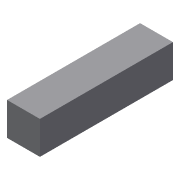
# Autodesk Inventor part: carbide_insert
Saved by Autodesk Inventor 2019 (Build 230136000, 136)
## iProperties
Created: 2023-02-17
Part Number: carbide_insert
Material: Generic
Document SubType Name: Modeling
Designer: prich
Density: 1 g/cm^3
Appearance: Default
Author: prich
Autodesk Inventor part; units mm, degrees
ref_plane "YZ Plane" through (0, 0, 0) normal (1, 0, 0) x (0, 1, 0)
ref_plane "XZ Plane" through (0, 0, 0) normal (0, 1, 0) x (-1, 0, 0)
ref_plane "XY Plane" through (0, 0, 0) normal (0, 0, 1) x (1, 0, 0)
sketch "Sketch1" plane through (0, 0, 0) normal (0, 0, 1) x (1, 0, 0)
  line L0 (0, 0) -> (1.6002, 0)
  line L1 (1.6002, 0) -> (1.6002, 1.6002)
  line L2 (1.6002, 1.6002) -> (0, 1.6002)
  line L3 (0, 1.6002) -> (0, 0)
  dimension "d0" = 1.6002
  dimension "d1" = 1.6002
  constraints: 8 end point, 2 parallel, 1 horizontal, 1 perpendicular
  measures "d0" distance of L1.end L2.end
  measures "d1" distance between parallel lines of L0 L2
extrude "Extrusion1" add sketch "Sketch1" along normal blind 6.477
equation "\"d1\" = d0"
body "Solid1"
